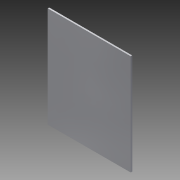
# Autodesk Inventor part: Base Plate
Saved by Autodesk Inventor 2015 (Build 190159000, 159)
## iProperties
Created: 2015-02-23
Part Number: Base Plate
Material: Aluminum 6061
Document SubType Name: Modeling
Designer: Andrew
Density: 2.7 g/cm^3
Appearance: Aluminum - Flat
Width: 140.000 mm
Author: Andrew
Autodesk Inventor part; units mm, degrees
ref_plane "YZ Plane" through (0, 0, 0) normal (1, 0, 0) x (0, 1, 0)
ref_plane "XZ Plane" through (0, 0, 0) normal (0, 1, 0) x (-1, 0, 0)
ref_plane "XY Plane" through (0, 0, 0) normal (0, 0, 1) x (1, 0, 0)
sketch "Sketch1" plane through (0, 0, 0) normal (0, 1, 0) x (-1, 0, 0)
  line L0 (70, 85) -> (-70, 85)
  line L1 (-70, 85) -> (-70, -85)
  line L2 (-70, -85) -> (70, -85)
  line L3 (70, -85) -> (70, 85)
  line L4 (0, -119) -> (0, 119) projected
  line L5 (-98, 0) -> (98, 0) projected
  point P0 (0, 0)
  dimension "Length" = 170
  dimension "Width" = 140
  constraints: 8 end point, 2 parallel, 1 horizontal, 1 perpendicular, 2 other
  measures "Length" distance of L2.end L0.start
  measures "Width" distance of L1.end L2.end
extrude "Extrusion1" add sketch "Sketch1" along normal blind 2.5
body "Solid1"
